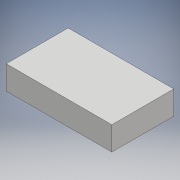
# Autodesk Inventor part: mbed
Saved by Autodesk Inventor 2017 (Build 210142000, 142)
## iProperties
Part Number: mbed
Material: 一般
Document SubType Name: Modeling
Designer: HISAAKI
Density: 1 g/cm^3
Appearance: 既定
Author: HISAAKI
Autodesk Inventor part; units mm, degrees
ref_plane "YZ Plane" through (0, 0, 0) normal (1, 0, 0) x (0, 1, 0)
ref_plane "XZ Plane" through (0, 0, 0) normal (0, 1, 0) x (-1, 0, 0)
ref_plane "XY Plane" through (0, 0, 0) normal (0, 0, 1) x (1, 0, 0)
sketch "スケッチ1" plane through (0, 0, 0) normal (0, 0, 1) x (1, 0, 0)
  line L0 (0, 0) -> (53.5, 0)
  line L1 (53.5, 0) -> (53.5, 31.4)
  line L2 (53.5, 31.4) -> (0, 31.4)
  line L3 (0, 31.4) -> (0, 0)
  dimension "d0" = 53.5
  dimension "d1" = 31.4
  constraints: 8 end point, 2 parallel, 1 horizontal, 1 perpendicular
  measures "d0" distance of L2.end L1.end
  measures "d1" distance of L1.end L0.end
extrude "押し出し1" add sketch "スケッチ1" along normal blind 12
